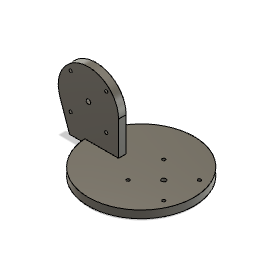
Link1 (Autodesk Fusion 360 design; units mm, degrees)
Autodesk Fusion 360 part; units mm, degrees
sketch "Sketch1" plane through (0, 0, 0) normal (0, 1, 0) x (1, 0, 0)
  circle A0 centre (0, 0) radius 70
  dimension "d1" = 140
  constraint coincident A0.centre origin
  measures "d1" diameter of A0
extrude "Extrude1" add sketch "Sketch1" along normal blind 10
sketch "Sketch2" plane through (0, 0, 0) normal (0, -1, 0) x (1, 0, 0)
  circle A0 centre (0, 0) radius 70
  circle A1 centre (0, 0) radius 65
  dimension "d4" = -5
extrude "Extrude2" add sketch "Sketch2" along normal blind 3 contours A1
sketch "Sketch3" plane through (0, 0, 0) normal (0, 0, 1) x (1, 0, 0)
  line L0 (-25, 55) -> (-25, 5)
  line L1 (-25, 5) -> (-90, 5)
  line L2 (-90, 5) -> (-102.7928, 41.8964)
  arc A0 (-25, 55) -> (-102.7928, 41.8964) centre (-65, 55) ccw
  dimension "d7" = 50
  dimension "d8" = 65
  dimension "d9" = 40
  dimension "d10" = 5
  dimension "d11" = 25
  constraint vertical L0
  constraint perpendicular L0 L1
  constraint tangent L2 A0
  constraint tangent L0 A0
  measures "d7" distance of L0.start L0.end
  measures "d8" distance of L0.end L1.end
  measures "d9" radius of A0
  measures "d10" vertical distance of origin L0.end
  measures "d11" horizontal distance of origin L0.end
extrude "Extrude3" add sketch "Sketch3" along normal mid plane 10
sketch "Sketch4" plane through (0, 10, 0) normal (0, 1, 0) x (-1, 0, 0)
  line L0 (25, 5) -> (69.8212, 5)
  arc A0 (69.8212, 5) -> (69.8212, -5) centre (0, 0) ccw
  line L1 (69.8212, -5) -> (25, -5)
  line L2 (25, -5) -> (25, 5)
  line L3 (-6.378, -23.622) -> (-53.622, -23.622)
  line L4 (-53.622, -23.622) -> (-53.622, 23.622)
  line L5 (-53.622, 23.622) -> (-6.378, 23.622)
  line L6 (-6.378, 23.622) -> (-6.378, -23.622)
  line L7 (-6.378, -23.622) -> (-53.622, 23.622) construction
  line L8 (-53.622, -23.622) -> (-6.378, 23.622) construction
  point P0 (-30, 0)
  dimension "d14" = 47.244
  dimension "d15" = 47.244
  dimension "d16" = 30
  constraint horizontal L3
  constraint perpendicular L3 L4
  constraint parallel L3 L5
  constraint parallel L4 L6
  constraint coincident L7 P0
  constraint coincident L8 P0
  constraint horizontal A0.centre P0
  measures "d14" distance of L4.end L5.end
  measures "d15" distance of L3.end L4.end
  measures "d16" distance of A0.centre P0
hole "Hole1" at (6.378, 10, 23.622) at (6.378, 10, -23.622) at (53.622, 10, -23.622) at (53.622, 10, 23.622) direction (0, -1, 0) diameter 4 depth 10 tip angle 118
hole "Hole2" at (30, 10, 0) direction (0, -1, 0) diameter 6 depth 15 tip angle 118
sketch "Sketch5" plane through (0, 0, 5) normal (0, 0, 1) x (1, 0, 0)
  line L0 (-69.8212, 10) -> (-25, 10)
  line L1 (-25, 10) -> (-25, 55)
  arc A0 (-25, 55) -> (-102.7928, 41.8964) centre (-65, 55) ccw
  line L2 (-102.7928, 41.8964) -> (-90, 5)
  line L3 (-90, 5) -> (-69.8212, 5)
  line L4 (-69.8212, 5) -> (-69.8212, 10)
  line L5 (-41.378, 78.622) -> (-88.622, 78.622)
  line L6 (-88.622, 78.622) -> (-88.622, 31.378)
  line L7 (-88.622, 31.378) -> (-41.378, 31.378)
  line L8 (-41.378, 31.378) -> (-41.378, 78.622)
  line L9 (-41.378, 78.622) -> (-88.622, 31.378) construction
  line L10 (-88.622, 78.622) -> (-41.378, 31.378) construction
  point P0 (-65, 55)
  dimension "d23" = 47.244
  dimension "d24" = 47.244
  constraint horizontal L5
  constraint perpendicular L5 L6
  constraint parallel L5 L7
  constraint parallel L6 L8
  constraint coincident L9 P0
  constraint coincident L10 P0
  constraint coincident P0 A0.centre
  measures "d23" distance of L6.end L7.end
  measures "d24" distance of L5.end L6.end
hole "Hole3" at (-88.622, 78.622, 5) at (-41.378, 78.622, 5) at (-41.378, 31.378, 5) at (-88.622, 31.378, 5) direction (0, 0, -1) diameter 4 depth 40 tip angle 118
hole "Hole4" at (-65, 55, 5) direction (0, 0, -1) diameter 6 depth 40 tip angle 118
